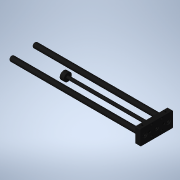
# Autodesk Inventor part: 529120 DFM-16-150-B-P-A-KF---(K)
Saved by Autodesk Inventor 2021 (Build 250183000, 183)
## iProperties
Created: 2025-06-19
Part Number: 529120 DFM-16-150-B-P-A-KF---(K)
Material: Generic
Catalog Web Link: www.cadenas.de
Description: DFM-B-(K)-Guide unit
Vendor: FESTO
Document SubType Name: Modeling
Designer: psAdmin
Manufacturer: FESTO
Mass: 64.4207 g
Surface Area: 269.956 cm^2
Volume: 64.4207 cm^3
Density: 1 g/cm^3
Appearance: PSOLRGB-128-128-128
Category: PARTsolutions
Company: FESTO
Title: 529120 DFM-16-150-B-P-A-KF---(K)
Author: Cadenas PARTsolutions
Comments: Guide unit
PSOL_IDENT_0: {$CADENAS_DATA/23d-libs/festo/parts/d/dfm/parts/dfm_b_k.prj},238 {VTYP=3D},{NB=529120 DFM-16-150-B-P
PSOL_IDENT_1: -A-KF---(K)},{LINA=529120 DFM-16-150-B-P-A-KF---(K)},{NN=DFM-B-(K)},{DATE=04.04.2025 09:37:05},{GEOM
PSOL_IDENT_2: DATE=04.04.2025 09:23:18},{VERSION=},{LINEID=550},{WBVAR=HUB,CUSH,F,JUST},{WBNUMERIC=HUB,CUSH,F,JUST
PSOL_IDENT_3: }  {NB=529120 DFM-16-150-B-P-A-KF---(K)},{LINA=529120 DFM-16-150-B-P-A-KF---(K)},{KT=1},{TNR=529120}
PSOL_IDENT_4: ,{TYP=DFM},{KDM=16},{HUB=150},{G=B},{CUSH=1},{F=2},{JUST=0},{VERS=1},{L16=0},{B1=67.000},{B2=65.000}
PSOL_IDENT_5: ,{B3=45.000},{B4=4.500},{B5=58.000},{B6=22.000},{B7=23.000},{B8=23.500},{B9=20.000},{B10=10.500},{B1
PSOL_IDENT_6: 1=46.000},{B12=9.500},{B13=46.000},{B14=21.300},{B15=24.400},{B16A=33.500},{B17A=0.000},{B18A=0.000}
PSOL_IDENT_7: ,{B19A=0.000},{B20=0.000},{B21=0.000},{B22=0.000},{D1=M 5},{D1P=5.000},{D1KDR=4.134},{D2=7.500},{D3=
PSOL_IDENT_8: 9.000},{D4=M 5},{D4P=5.000},{D4KDR=4.134},{D5=5.000},{D6=4.3},{D6P=4.300},{D6KDR=3.242},{D7=10},{D7G
PSOL_IDENT_9: F=12.000},{D7KF=10.000},{D8=5.000},{D9=M 4},{D9P=4.000},{D9KDR=3.242},{D10=6.000},{FN=2},{FT=-KF},{E
PSOL_IDENT_10: 1=M 5},{EEMM=5.000},{EEKDR=4.134},{H1=32.000},{H2=30.000},{H3=26.500},{H4=4.000},{H5=24.000},{H6=4.0
PSOL_IDENT_11: 00},{H7=24.000},{H8=16.000},{H9=7.400},{H10=20.000},{H11=16.000},{H12A=16.000},{H13A=0.000},{H14A=16
PSOL_IDENT_12: .000},{L1=264},{L2=58.000},{L3=10.000},{L4=12.000},{L5=9.800},{L6A=9.300},{L7=34},{L8=22.000},{L9=40
PSOL_IDENT_13: },{L10=34.000},{L11=120},{L12=5.000},{L13A=4.000},{L14=0},{L15=0},{T1=12.000},{T2=4.600},{T3=2.100},
PSOL_IDENT_14: {T4=10.000},{T5=1.200},{T6=0.000},{T7=0.000},{T8=0.000},{T9=0.000},{T9L=0.000},{SW1=10.000},{SW2=10.
PSOL_IDENT_15: 000},{SW3=17.000},{SW4=0.000},{SW4D=0.000},{SW4KDR=0.000},{SW4M=0.000},{SW5=0.000},{SW6=0.000},{SW7=
PSOL_IDENT_16: 0.000},{SW8=0.000},{SW9=0.000},{SW10=0.000},{SW2D=6.000},{SW2T=4.000},{ZZ=0},{MOD=1},{BR=0.000},{HUB
PSOL_IDENT_17: 1=[10:200]},{YB1=0.000},{YD1=0.000},{YD2=0.000},{YD3=0.000},{YD4=0.000},{YL1=0.000},{YL2=0.000},{YL3=
PSOL_IDENT_18: 0.000},{YL4=0.000},{YL5=0.000},{YL6=0.000},{YL7=0.000},{YL14=0.000},{L14A=107.900},{L14Y=0.000},{L15
PSOL_IDENT_19: A=0.000},{L15Y=0.000},{L16A=107.900},{L16Y=0.000},{CUSHT=-P},{CUSHN=1},{JT=},{B16=0},{B17=0},{B18=0}
PSOL_IDENT_20: ,{B19=0},{H12=0},{H13=0},{H14=0},{L6=0},{L13=0},{PPV1= 1, 'P', 2, 'PPV'},{PPV2= 1, 'P', 2, 'PPV'},{P
PSOL_IDENT_21: PV= 1, 'P', 2, 'PPV'},{JU= 0, '-', 1, 'AJ', 2, 'EJ', 3, 'AJ+EJ'},{FE= 0, '-', 1, 'AJ', 2, 'EJ', 3, '
PSOL_IDENT_22: AJ+EJ'},{FE1= 0, '-'},{VER=1.000},{GH1=8.000},{GH2=12.000},{DH1=0.000},{DH2=0.000},{VERO=2},{A1=0.00
PSOL_IDENT_23: 0},{A2=0.000},{A3=0.000},{A4=0.000},{A5=0.000},{A6=0.000},{A7D=0.000},{I1=28.000},{A8=0.000},{A9=1.4
PSOL_IDENT_24: 00},{HR1=0.000},{LR1=0.000},{LR2=0.000},{HR2=0.000},{DEG=0.000},{DR1=0.000},{DR2=0.000},{D17=18.000}
PSOL_IDENT_25: ,{D18=10.000},{H15=4.000},{D19=0.000},{D12=6.000},{D12P=1.000},{SCA=0.000},{D20=0.000},{B23=0.000},{
PSOL_IDENT_26: B24=0.000},{D21=0.000},{R1=0.000}
NB: 529120 DFM-16-150-B-P-A-KF---(K)
NN: DFM-B-(K)
NT: Guide unit
NBSYN: $TNR. $TYP.-$KDM.-$HUB.-$G.$CUSHT.-A$FT.$JT.---(K)
LINA: 529120 DFM-16-150-B-P-A-KF---(K)
CATALOG: Festo
TNR: 529120
TYP: DFM
KDM: 16
HUB: 150
G: B
CUSH: P
F: KF
JUST: -
L16: 0
B1: 67
B2: 65
B3: 45
B4: 4.5
B5: 58
B6: 22
B7: 23
B8: 23.5
B9: 20
B10: 10.5
B11: 46
B12: 9.5
B13: 46
B14: 21.3
B15: 24.4
B16A: 33.5
B17A: 0
B18A: 0
B19A: 0
B20: 0
B21: 0
B22: 0
D1: M 5
D1P: 5
D1KDR: 4.134
D2: 7.5
D3: 9
D4: M 5
D4P: 5
D4KDR: 4.134
D5: 5
D6: 4.3
D6P: 4.3
D6KDR: 3.242
D7GF: 12
D7KF: 10
D8: 5
D9: M 4
D9P: 4
D9KDR: 3.242
D10: 6
E1: M 5
EEKDR: 4.134
H1: 32
H2: 30
H3: 26.5
H4: 4
H5: 24
H6: 4
H7: 24
H8: 16
H9: 7.4
H10: 20
H11: 16
H12A: 16
H13A: 0
H14A: 16
L2: 58
L3: 10
L4: 12
L5: 9.8
L6A: 9.3
L8: 22
L10: 34
L12: 5
L13A: 4
T1: 12
T2: 4.6
T3: 2.1
T4: 10
T5: 1.2
T6: 0
T7: 0
T8: 0
T9: 0
T9L: 0
SW1: 10
SW2: 10
SW3: 17
SW4: 0
SW4D: 0
SW4KDR: 0
SW4M: 0
SW5: 0
SW6: 0
SW7: 0
SW8: 0
SW9: 0
SW10: 0
SW2D: 6
SW2T: 4
BR: 0
HUB1: [10:200]
YB1: 0
YD1: 0
YD2: 0
YD3: 0
YD4: 0
YL1: 0
YL2: 0
YL3: 0
YL4: 0
YL5: 0
YL6: 0
YL7: 0
YL14: 0
L14A: 107.9
L14Y: 0
L15A: 0
L15Y: 0
L16A: 107.9
L16Y: 0
PPV1: 1, 'P', 2, 'PPV'
PPV2: 1, 'P', 2, 'PPV'
FE: 0, '-', 1, 'AJ', 2, 'EJ', 3, 'AJ+EJ'
FE1: 0, '-'
VER: 1
GH1: 8
GH2: 12
DH1: 0
DH2: 0
A1: 0
A2: 0
A3: 0
A4: 0
A5: 0
A6: 0
A7D: 0
I1: 28
A8: 0
A9: 1.4
HR1: 0
LR1: 0
LR2: 0
HR2: 0
DEG: 0
DR1: 0
DR2: 0
D17: 18
D18: 10
H15: 4
D19: 0
D12: 6
D12P: 1
SCA: 0
D20: 0
B23: 0
B24: 0
D21: 0
R1: 0
SUPPLIER: FESTO
ARTICLENO: 529120 DFM-16-150-B-P-A-KF---(K)
BOMINFO: 529120 DFM-16-150-B-P-A-KF---(K)
CREATOR: CADENAS GmbH
Autodesk Inventor part; units mm, degrees
sketch "Skizze_1" plane through (12, 0, 0) normal (1, 0, 0) x (0, 0, -1)
  line L0 (-32.5, -14) -> (-31.5, -15)
  line L1 (-31.5, -15) -> (31.5, -15)
  line L2 (31.5, -15) -> (32.5, -14)
  line L3 (32.5, -14) -> (32.5, 14)
  line L4 (32.5, 14) -> (31.5, 15)
  line L5 (31.5, 15) -> (-31.5, 15)
  line L6 (-31.5, 15) -> (-32.5, 14)
  line L7 (-32.5, 14) -> (-32.5, -14)
  constraints: 16 end point
extrude "Extrusion1" add sketch "Skizze_1" against normal blind 10
sketch "Skizze_2" plane through (0, 0, 0) normal (0, 1, 0) x (1, 0, 0)
  line L0 (-252, -23) -> (2, -23)
  line L1 (2, -23) -> (2, -28)
  line L2 (2, -28) -> (-251, -28)
  line L3 (-251, -28) -> (-252, -27.4226)
  line L4 (-252, -27.4226) -> (-252, -23)
  line L5 (-252, -23) -> (2, -23)
  constraints: 12 end point
sketch "Skizze_3" plane through (0, 0, 0) normal (0, 1, 0) x (1, 0, 0)
  line L0 (-252, 23) -> (2, 23)
  line L1 (2, 23) -> (2, 18)
  line L2 (2, 18) -> (-251, 18)
  line L3 (-251, 18) -> (-252, 18.5774)
  line L4 (-252, 18.5774) -> (-252, 23)
  line L5 (-252, 23) -> (2, 23)
  constraints: 12 end point
sketch "Skizze_4" plane through (0, -8.6, 0) normal (0, 1, 0) x (1, 0, 0)
  line L0 (12, -10) -> (2, -10)
  line L1 (2, -10) -> (2, -7.5)
  line L2 (2, -7.5) -> (2.433, -7.933)
  line L3 (2.433, -7.933) -> (11.567, -7.933)
  line L4 (11.567, -7.933) -> (12, -7.5)
  line L5 (12, -7.5) -> (12, -10)
  line L6 (12, -10) -> (2, -10)
  constraints: 14 end point
revolve "Revolution1" cut sketch "Skizze_4" angle 360 about axis through (12, -8.6, 10) along (1, 0, 0)
thread "Thread1" size "M5x0.8" class "6H" standard "ISO Metric profile" full length
sketch "Skizze_5" plane through (0, -8.6, 0) normal (0, 1, 0) x (1, 0, 0)
  line L0 (12, 10) -> (2, 10)
  line L1 (2, 10) -> (2, 12.5)
  line L2 (2, 12.5) -> (2.433, 12.067)
  line L3 (2.433, 12.067) -> (11.567, 12.067)
  line L4 (11.567, 12.067) -> (12, 12.5)
  line L5 (12, 12.5) -> (12, 10)
  line L6 (12, 10) -> (2, 10)
  constraints: 14 end point
revolve "Revolution2" cut sketch "Skizze_5" angle 360 about axis through (12, -8.6, -10) along (1, 0, 0)
thread "Thread2" size "M5x0.8" class "6H" standard "ISO Metric profile" full length
sketch "Skizze_6" plane through (0, 11.4, 0) normal (0, 1, 0) x (1, 0, 0)
  line L0 (12, -10) -> (2, -10)
  line L1 (2, -10) -> (2, -7.5)
  line L2 (2, -7.5) -> (2.433, -7.933)
  line L3 (2.433, -7.933) -> (11.567, -7.933)
  line L4 (11.567, -7.933) -> (12, -7.5)
  line L5 (12, -7.5) -> (12, -10)
  line L6 (12, -10) -> (2, -10)
  constraints: 14 end point
revolve "Revolution3" cut sketch "Skizze_6" angle 360 about axis through (12, 11.4, 10) along (1, 0, 0)
thread "Thread3" size "M5x0.8" class "6H" standard "ISO Metric profile" full length
sketch "Skizze_7" plane through (0, 11.4, 0) normal (0, 1, 0) x (1, 0, 0)
  line L0 (12, 10) -> (2, 10)
  line L1 (2, 10) -> (2, 12.5)
  line L2 (2, 12.5) -> (2.433, 12.067)
  line L3 (2.433, 12.067) -> (11.567, 12.067)
  line L4 (11.567, 12.067) -> (12, 12.5)
  line L5 (12, 12.5) -> (12, 10)
  line L6 (12, 10) -> (2, 10)
  constraints: 14 end point
revolve "Revolution4" cut sketch "Skizze_7" angle 360 about axis through (12, 11.4, -10) along (1, 0, 0)
thread "Thread4" size "M5x0.8" class "6H" standard "ISO Metric profile" full length
sketch "Skizze_8" plane through (0, 0, 0) normal (0, 0, 1) x (1, 0, 0)
  line L0 (2, 0) -> (-171.95, 0)
  line L1 (-171.95, 0) -> (-171.95, 8)
  line L2 (-171.95, 8) -> (-163.95, 8)
  line L3 (-163.95, 8) -> (-163.95, 3)
  line L4 (-163.95, 3) -> (2, 3)
  line L5 (2, 3) -> (2, 0)
  line L6 (2, 0) -> (-171.95, 0)
  constraints: 14 end point
revolve "Revolution5" add sketch "Skizze_8" angle 360 about axis through (2, 0, 0) along (1, 0, 0)
sketch "Sketch9" plane through (12, 15, 31.5) normal (0, 1, 0) x (1, 0, 0)
  point P0 (-5, 8.5)
hole "Hole1" at (7, 15, 23) direction (0, -1, 0) diameter 3.242 depth 15 countersink diameter 4 countersink angle 90 thread size "M4x0.7" class "6H" standard "ISO Metric profile"
sketch "Sketch10" plane through (12, 15, 31.5) normal (0, 1, 0) x (1, 0, 0)
  point P0 (-5, 54.5)
hole "Hole2" at (7, 15, -23) direction (0, -1, 0) diameter 3.242 depth 15 countersink diameter 4 countersink angle 90 thread size "M4x0.7" class "6H" standard "ISO Metric profile"
revolve "Revolution6" add sketch "Skizze_2" angle 360 about axis through (-252, 0, 23) along (-1, 0, 0)
revolve "Revolution7" add sketch "Skizze_3" angle 360 about axis through (-252, 0, -23) along (-1, 0, 0)
sketch "Sketch11" plane through (12, 0, 0) normal (1, 0, 0) x (0, 0, -1)
  point P0 (14, 1.4)
hole "Hole3" at (12, 1.4, -14) direction (-1, 0, 0) diameter 5 depth 1 tip angle 120
sketch "Sketch12" plane through (12, 0, 0) normal (1, 0, 0) x (0, 0, -1)
  point P0 (-14, 1.4)
hole "Hole4" at (12, 1.4, 14) direction (-1, 0, 0) diameter 5 depth 1 tip angle 120
sketch "Sketch_4" plane through (0, 0, 0) normal (0, 1, 0) x (1, 0, 0)
  line L0 (12, 23) -> (11.65, 23)
  line L1 (11.65, 23) -> (11.65, 26.4725)
  arc A0 (11.65, 26.4725) -> (11.1936, 26.9706) centre (11.15, 26.4725) ccw
  line L2 (11.1936, 26.9706) -> (8, 27.25)
  line L3 (8, 27.25) -> (8, 28)
  line L4 (8, 28) -> (12, 28)
  line L5 (12, 28) -> (12, 23)
  line L6 (12, 23) -> (11.65, 23)
  constraints: 14 end point, 2 point on circle, 1 centre point
revolve "Revolution8" cut sketch "Sketch_4" angle 360 about axis through (12, 0, -23) along (1, 0, 0)
sketch "Sketch_6" plane through (0, 0, 0) normal (0, 1, 0) x (1, 0, 0)
  line L0 (12, -23) -> (11.65, -23)
  line L1 (11.65, -23) -> (11.65, -19.5275)
  arc A0 (11.65, -19.5275) -> (11.1936, -19.0294) centre (11.15, -19.5275) ccw
  line L2 (11.1936, -19.0294) -> (8, -18.75)
  line L3 (8, -18.75) -> (8, -18)
  line L4 (8, -18) -> (12, -18)
  line L5 (12, -18) -> (12, -23)
  line L6 (12, -23) -> (11.65, -23)
  constraints: 14 end point, 2 point on circle, 1 centre point
revolve "Revolution9" cut sketch "Sketch_6" angle 360 about axis through (12, 0, 23) along (1, 0, 0)
sketch "Sketch_7" plane through (11.65, 0, 23) normal (1, 0, 0) x (0, 0, -1)
  arc A0 (-1.8677, -0.5727) -> (-1.4298, -1.3311) centre (-1.5588, -0.9) ccw
  arc A1 (-0.4379, -1.9038) -> (-1.4298, -1.3311) centre (-1.2041, -2.0855) ccw
  arc A2 (-0.4379, -1.9038) -> (0.4379, -1.9038) centre (0, -1.8) ccw
  arc A3 (1.4298, -1.3311) -> (0.4379, -1.9038) centre (1.2041, -2.0855) ccw
  arc A4 (1.4298, -1.3311) -> (1.8677, -0.5727) centre (1.5588, -0.9) ccw
  arc A5 (1.8677, 0.5727) -> (1.8677, -0.5727) centre (2.4082, 0) ccw
  arc A6 (1.8677, 0.5727) -> (1.4298, 1.3311) centre (1.5588, 0.9) ccw
  arc A7 (0.4379, 1.9038) -> (1.4298, 1.3311) centre (1.2041, 2.0855) ccw
  arc A8 (0.4379, 1.9038) -> (-0.4379, 1.9038) centre (0, 1.8) ccw
  arc A9 (-1.4298, 1.3311) -> (-0.4379, 1.9038) centre (-1.2041, 2.0855) ccw
  arc A10 (-1.4298, 1.3311) -> (-1.8677, 0.5727) centre (-1.5588, 0.9) ccw
  arc A11 (-1.8677, -0.5727) -> (-1.8677, 0.5727) centre (-2.4082, 0) ccw
  constraints: 24 point on circle, 12 centre point
extrude "Extrusion2" cut sketch "Sketch_7" against normal blind 2.48
sketch "Sketch_8" plane through (11.65, 0, -23) normal (1, 0, 0) x (0, 0, -1)
  arc A0 (-1.8677, -0.5727) -> (-1.4298, -1.3311) centre (-1.5588, -0.9) ccw
  arc A1 (-0.4379, -1.9038) -> (-1.4298, -1.3311) centre (-1.2041, -2.0855) ccw
  arc A2 (-0.4379, -1.9038) -> (0.4379, -1.9038) centre (0, -1.8) ccw
  arc A3 (1.4298, -1.3311) -> (0.4379, -1.9038) centre (1.2041, -2.0855) ccw
  arc A4 (1.4298, -1.3311) -> (1.8677, -0.5727) centre (1.5588, -0.9) ccw
  arc A5 (1.8677, 0.5727) -> (1.8677, -0.5727) centre (2.4082, 0) ccw
  arc A6 (1.8677, 0.5727) -> (1.4298, 1.3311) centre (1.5588, 0.9) ccw
  arc A7 (0.4379, 1.9038) -> (1.4298, 1.3311) centre (1.2041, 2.0855) ccw
  arc A8 (0.4379, 1.9038) -> (-0.4379, 1.9038) centre (0, 1.8) ccw
  arc A9 (-1.4298, 1.3311) -> (-0.4379, 1.9038) centre (-1.2041, 2.0855) ccw
  arc A10 (-1.4298, 1.3311) -> (-1.8677, 0.5727) centre (-1.5588, 0.9) ccw
  arc A11 (-1.8677, -0.5727) -> (-1.8677, 0.5727) centre (-2.4082, 0) ccw
  constraints: 24 point on circle, 12 centre point
extrude "Extrusion3" cut sketch "Sketch_8" against normal blind 2.48
sketch "Sketch_9" plane through (0, 0, 0) normal (0, 0, 1) x (1, 0, 0)
  line L0 (12, 0) -> (9.868, 0)
  line L1 (9.868, 0) -> (11.6, 1.732)
  line L2 (11.6, 1.732) -> (11.6, 3.1)
  arc A0 (11.6, 3.1) -> (11.2, 3.5) centre (11.2, 3.1) ccw
  line L3 (11.2, 3.5) -> (7.6, 3.5)
  line L4 (7.6, 3.5) -> (7.6, 4)
  line L5 (7.6, 4) -> (12, 4)
  line L6 (12, 4) -> (12, 0)
  line L7 (12, 0) -> (9.868, 0)
  constraints: 16 end point, 2 point on circle, 1 centre point
revolve "Revolution10" cut sketch "Sketch_9" angle 360 about axis through (12, 0, 0) along (1, 0, 0)
sketch "Sketch_10" plane through (11.6, 0, 0) normal (1, 0, 0) x (0, 1, 0)
  line L0 (-1.5, -0.866) -> (0, -1.7321)
  line L1 (0, -1.7321) -> (1.5, -0.866)
  line L2 (1.5, -0.866) -> (1.5, 0.866)
  line L3 (1.5, 0.866) -> (0, 1.7321)
  line L4 (0, 1.7321) -> (-1.5, 0.866)
  line L5 (-1.5, 0.866) -> (-1.5, -0.866)
  constraints: 12 end point
extrude "Extrusion4" cut sketch "Sketch_10" against normal blind 2
ref_plane "HUELSE3_1_XY" through (11, 1.4, -14) normal (1, 0, 0) x (0, 0, -1)
ref_plane "HUELSE3_1_YZ" through (11, 1.4, -14) normal (0, 0, -1) x (0, 1, 0)
ref_plane "HUELSE3_1_ZX" through (11, 1.4, -14) normal (0, 1, 0) x (1, 0, 0)
ref_plane "HUELSE3_2_XY" through (11, 1.4, 14) normal (1, 0, 0) x (0, 0, -1)
ref_plane "HUELSE3_2_YZ" through (11, 1.4, 14) normal (0, 0, -1) x (0, 1, 0)
ref_plane "HUELSE3_2_ZX" through (11, 1.4, 14) normal (0, 1, 0) x (1, 0, 0)
ref_plane "kolben_dfm_XY" through (0, 0, 0) normal (-1, 0, 0) x (0, 0, -1)
ref_plane "kolben_dfm_YZ" through (0, 0, 0) normal (0, 0, -1) x (0, -1, 0)
ref_plane "kolben_dfm_ZX" through (0, 0, 0) normal (0, -1, 0) x (-1, 0, 0)
body "Solid1"
